9ee541ba-d0e4-4538-9089-a28fc8009398 (Autodesk Fusion 360 design; units mm, degrees)
Autodesk Fusion 360 part; units mm, degrees
note: some values were not read from the file. Set by a fixed rule: which sketch regions a step uses.
sketch "Sketch1" plane through (0, 0, 0) normal (0, 1, 0) x (1, 0, 0)
  circle A0 centre (0, 0) radius 6.35
  circle A1 centre (0, 0) radius 7.366
  circle A2 centre (0, 0) radius 5.2917
  circle A3 centre (0, 0) radius 5.967
  arc A4 (7.3471, -0.527) -> (-6.7515, -2.9454) centre (0, 0) ccw
  circle A5 centre (0, 0) radius 1.9844
  line L0 (0, 0) -> (7.366, 0) construction
  line L1 (0, 0) -> (-0.5201, -5.9443)
  line L2 (0, 0) -> (-1.0362, -5.8764)
  line L3 (0, 0) -> (-1.5444, -5.7637)
  line L4 (0, 0) -> (-2.0409, -5.6072)
  line L5 (0, 0) -> (-2.5218, -5.408)
  line L6 (0, 0) -> (-2.9835, -5.1676)
  line L7 (0, 0) -> (-3.4226, -4.8879)
  line L8 (-0.5201, -5.9443) -> (-0.0013, -5.9897) construction
  line L9 (-1.0362, -5.8764) -> (-0.0105, -6.0572) construction
  line L10 (-1.5444, -5.7637) -> (-0.0354, -6.168) construction
  line L11 (-2.0409, -5.6072) -> (-0.0836, -6.3196) construction
  line L12 (-2.5218, -5.408) -> (-0.1621, -6.5083) construction
  line L13 (-2.9835, -5.1676) -> (-0.2778, -6.7298) construction
  line L14 (-3.4226, -4.8879) -> (-0.4367, -6.9786) construction
  line L15 (0, 0) -> (-3.8355, -4.571)
  line L16 (-3.8355, -4.571) -> (-0.6444, -7.2487) construction
  line L17 (0, 0) -> (-4.2193, -4.2193)
  line L18 (-4.2193, -4.2193) -> (-0.9055, -7.5332) construction
  spline S0 degree 5 poles (-0.9055, -7.5332) (-0.8962, -7.5235) (-0.8778, -7.504) (-0.8503, -7.475) (-0.8141, -7.4367) (-0.7697, -7.3892) (-0.7263, -7.3419) (-0.6841, -7.2948) (-0.6432, -7.2478) (-0.6037, -7.2007) (-0.5658, -7.1536) (-0.5293, -7.1065) (-0.4942, -7.0596) (-0.4605, -7.0129) (-0.4281, -6.9665) (-0.3968, -6.9205) (-0.3669, -6.875) (-0.3381, -6.83) (-0.3106, -6.7855) (-0.2843, -6.7415) (-0.2594, -6.698) (-0.2358, -6.6552) (-0.2134, -6.613) (-0.1923, -6.5715) (-0.1725, -6.5308) (-0.1539, -6.4909) (-0.1364, -6.4518) (-0.1202, -6.4138) (-0.1051, -6.3767) (-0.0912, -6.3407) (-0.0784, -6.3058) (-0.0668, -6.2721) (-0.0562, -6.2397) (-0.0467, -6.2086) (-0.0383, -6.1789) (-0.0308, -6.1507) (-0.0242, -6.1241) (-0.0186, -6.0992) (-0.0139, -6.076) (-0.01, -6.0547) (-0.0069, -6.0353) (-0.0045, -6.018) (-0.0027, -6.0029) (-0.0013, -5.9903) (-0.0004, -5.9802) (0.0001, -5.9728) (0.0003, -5.9691) (0.0002, -5.9676) (0.0001, -5.9671) (0, -5.967) knots 0 0 0 0 0 0 0.022222 0.044444 0.066667 0.088889 0.111111 0.133333 0.155556 0.177778 0.2 0.222222 0.244444 0.266667 0.288889 0.311111 0.333333 0.355556 0.377778 0.4 0.422222 0.444444 0.466667 0.488889 0.511111 0.533333 0.555556 0.577778 0.6 0.622222 0.644444 0.666667 0.688889 0.711111 0.733333 0.755556 0.777778 0.8 0.822222 0.844444 0.866667 0.888889 0.911111 0.933333 0.955556 0.977778 1 1 1 1 1 1
  line L19 (-1.012, -7.6454) -> (-0.7989, -7.421)
  line L20 (0.0091, -5.9765) -> (-0.0091, -5.9576)
  line L21 (-0.0946, -6.3493) -> (0, 0)
  line L22 (0, 0) -> (-0.8866, -6.0377) construction
  line L23 (0, -5.967) -> (0, 0) construction
  spline S1 degree 5 poles (0, -5.967) (0, -5.9285) (0, -5.8556) (0, -5.7592) (0, -5.6519) (0, -5.5361) (0, -5.4448) (0, -5.3711) (0, -5.3187) (0, -5.2917) knots 0 0 0 0 0 0 0.2 0.4 0.6 0.8 1 1 1 1 1 1
  spline S2 degree 5 poles (-1.7155, -5.7151) (-1.7044, -5.6782) (-1.6834, -5.6084) (-1.6557, -5.516) (-1.6249, -5.4133) (-1.5916, -5.3024) (-1.5653, -5.215) (-1.5441, -5.1443) (-1.5291, -5.0941) (-1.5213, -5.0683) knots 0 0 0 0 0 0 0.2 0.4 0.6 0.8 1 1 1 1 1 1
  line L24 (0, -6.0408) -> (0, -5.8933)
  line L25 (0, -5.3433) -> (0, -5.24)
  line L26 (-1.7367, -5.7858) -> (-1.6943, -5.6445)
  line L27 (-1.5362, -5.1178) -> (-1.5064, -5.0188)
  spline S3 degree 5 poles (-1.2985, -7.4755) (-1.3045, -7.4635) (-1.3166, -7.4396) (-1.3346, -7.4039) (-1.3582, -7.3568) (-1.3871, -7.2985) (-1.4151, -7.2408) (-1.442, -7.1835) (-1.4676, -7.1267) (-1.4919, -7.0703) (-1.5147, -7.0142) (-1.5361, -6.9587) (-1.5562, -6.9036) (-1.5751, -6.8492) (-1.5928, -6.7954) (-1.6095, -6.7424) (-1.6251, -6.6902) (-1.6397, -6.6388) (-1.6533, -6.5883) (-1.6658, -6.5386) (-1.6772, -6.4899) (-1.6875, -6.442) (-1.6968, -6.3952) (-1.705, -6.3494) (-1.7123, -6.3046) (-1.7187, -6.2611) (-1.7242, -6.2187) (-1.7288, -6.1776) (-1.7326, -6.1377) (-1.7355, -6.0992) (-1.7377, -6.0622) (-1.7392, -6.0265) (-1.74, -5.9924) (-1.7401, -5.9599) (-1.7397, -5.9291) (-1.7388, -5.8999) (-1.7374, -5.8726) (-1.7357, -5.8471) (-1.7335, -5.8235) (-1.7311, -5.8019) (-1.7285, -5.7825) (-1.7258, -5.7652) (-1.7232, -5.7503) (-1.7209, -5.7378) (-1.7189, -5.7279) (-1.7173, -5.7206) (-1.7163, -5.717) (-1.7158, -5.7156) (-1.7156, -5.7152) (-1.7155, -5.7151) knots 0 0 0 0 0 0 0.022222 0.044444 0.066667 0.088889 0.111111 0.133333 0.155556 0.177778 0.2 0.222222 0.244444 0.266667 0.288889 0.311111 0.333333 0.355556 0.377778 0.4 0.422222 0.444444 0.466667 0.488889 0.511111 0.533333 0.555556 0.577778 0.6 0.622222 0.644444 0.666667 0.688889 0.711111 0.733333 0.755556 0.777778 0.8 0.822222 0.844444 0.866667 0.888889 0.911111 0.933333 0.955556 0.977778 1 1 1 1 1 1
  line L28 (-1.2286, -7.6136) -> (-1.3683, -7.3374)
  line L29 (-1.7269, -5.7215) -> (-1.7041, -5.7087)
  point P0 (-0.0946, -6.3493)
  point P1 (0, -5.2917)
  point P2 (-1.4668, -7.128)
  point P3 (-1.588, -6.8096)
  point P4 (-1.6687, -6.5255)
  point P5 (-1.7158, -6.2802)
  point P6 (-1.7368, -6.0768)
  point P7 (-1.7393, -5.9178)
  point P8 (-1.7313, -5.8046)
  point P9 (-1.7207, -5.7372)
  point P10 (-1.5213, -5.0683)
  dimension "d2" = 14.732
  dimension "id" = 10.5833
  dimension "BaseDiameter" = 11.9341
  dimension "d1" = 3.9688
  dimension "d34" = 5
  dimension "d35" = 5
  dimension "d36" = 5
  dimension "d37" = 5
  dimension "d38" = 5
  dimension "d39" = 5
  dimension "d41" = 0.5207
  dimension "d42" = 1.0414
  dimension "d43" = 1.5622
  dimension "d44" = 2.0829
  dimension "d45" = 2.6036
  dimension "d46" = 3.1243
  dimension "d47" = 3.6451
  dimension "d48" = 5
  dimension "d49" = 4.1658
  dimension "d50" = 5
  dimension "d51" = 4.6865
  dimension "d55" = 7.5
  dimension "d60" = 5
  constraint coincident A0.centre A1.centre
  constraint concentric A0 A2
  constraint coincident A1 A4.end
  constraint horizontal L0
  constraint coincident A4 L0.end
  constraint coincident A3 S0.end
  constraint coincident A3 L1.end
  constraint coincident A3 L2.end
  constraint coincident A3 L3.end
  constraint coincident A3 L4.end
  constraint coincident A3 L5.end
  constraint coincident A3 L6.end
  constraint coincident A3 L7.end
  constraint vertical A0.centre S0.end
  constraint tangent A3 L8
  constraint tangent A3 L9
  constraint tangent A3 L10
  constraint tangent A3 L11
  constraint tangent A3 L12
  constraint tangent A3 L13
  constraint tangent A3 L14
  constraint coincident A3 L15.end
  constraint tangent A3 L16
  constraint coincident A3 L17.end
  constraint tangent A3 L18
  constraint midpoint L18.end L19
  constraint midpoint S0.end L20
  constraint coincident A0 P0
  constraint coincident S0 P0
  constraint coincident P0 L21.start
  constraint coincident L23 P1
  constraint coincident A2 P1
  constraint coincident P1 S1.end
  constraint midpoint S0.end L24
  constraint midpoint P1 L25
  constraint symmetric S0.end L22 S2.start
  constraint symmetric L8.end L22 P9
  constraint symmetric L9.end L22 P8
  constraint symmetric L10.end L22 P7
  constraint symmetric L11.end L22 P6
  constraint symmetric L12.end L22 P5
  constraint symmetric L13.end L22 P4
  constraint symmetric L14.end L22 P3
  constraint symmetric L16.end L22 P2
  constraint symmetric L18.end L22 S3.start
  constraint symmetric L19.start L22 L28.start
  constraint symmetric L19.end L22 L28.end
  constraint symmetric L20.start L22 L29.start
  constraint symmetric L20.end L22 L29.end
  constraint symmetric L22 P1 P10
  constraint symmetric L22 L24.start L26.start
  constraint symmetric L22 L24.end L26.end
  constraint symmetric L22 L25.start L27.start
  constraint symmetric L22 L25.end L27.end
  constraint vertical L24
  constraint vertical L25
  measures "d2" diameter of A1
  measures "id" diameter of A2
  measures "BaseDiameter" diameter of A3
  measures "d1" diameter of A5
  measures "d34" angle of L1 L2
  measures "d35" angle of L2 L3
  measures "d36" angle of L3 L4
  measures "d37" angle of L4 L5
  measures "d38" angle of L5 L6
  measures "d39" angle of L6 L7
  measures "d41" distance of L1.end L8.end
  measures "d42" distance of L2.end L9.end
  measures "d43" distance of L3.end L10.end
  measures "d44" distance of L4.end L11.end
  measures "d45" distance of L5.end L12.end
  measures "d46" distance of L6.end L13.end
  measures "d47" distance of L7.end L14.end
  measures "d48" angle of L7 L15
  measures "d49" distance of L15.end L16.end
  measures "d50" angle of L15 L17
  measures "d51" distance of L17.end L18.end
  measures "d55" angle of L21 L22
  measures "d60" angle of L1 L23
extrude "Extrude1" add sketch "Sketch1" along normal blind 304.8 contours A0 A1 S0 S3 | A3 S0 L21 | A0 A3 L21 S3 | A2 A3 L21 S1 L24 L25 | A2 A3 L1 L21 | A2 A3 L3 S2 L26 L27 | A2 A3 L1 L2 | A2 A3 L2 L3 makes body 1
pattern_circular "C-Pattern2" count 12 over 360 about axis through (0, 1.75, 0) along (0, 1, 0) of bodies 1 makes body 2 at (1.3828, 101.6, 5.1078) makes body 3 at (3.7515, 101.6, 3.7321) makes body 4 at (5.1149, 101.6, 1.3563) makes body 5 at (5.1078, 101.6, -1.3828) makes body 6 at (3.7321, 101.6, -3.7515) makes body 7 at (1.3563, 101.6, -5.1149) makes body 8 at (-1.3828, 101.6, -5.1078) makes body 9 at (-3.7515, 101.6, -3.7321) makes body 10 at (-5.1149, 101.6, -1.3563) makes body 11 at (-5.1078, 101.6, 1.3828) makes body 12 at (-3.7321, 101.6, 3.7515)
extrude "Extrude2" add sketch "Sketch1" along normal blind 304.8 contours A2 A5 L17 L21 | A2 A5 L1 L21 | A2 A5 L1 L2 | A2 A5 L3 L4 | A2 A5 L4 L5 | A2 A5 L2 L3 | A2 A5 L15 L17 | A2 A5 L5 L6 | A2 A5 L7 L15 | A2 A5 L6 L7 bodies 1 2 3 4 5 6 7 8 9 10 11 12
ref_plane "WorkPlane1" through (6.2747, 152.4, -0.8261) normal (0.130526, 0, 0.991445) x (0.991445, 0, -0.130526)
fillet "Fillet1" [suppressed]
mirror "Mirror3" [suppressed]
pattern_circular "C-Pattern1" [suppressed]
equation "d = 0.5 in"
equation "OutsideDiameter = d2"
equation "PitchDiameter = d"
equation "id = PitchDiameter - 2 * ( PitchDiameter / TeethNumber )"
equation "BaseDiameter = PitchDiameter * cos(20 deg)"
equation "Length = 12 in"
equation "t = 12"
equation "ShaftDiameter = d1"
equation "TeethNumber = t"
equation "Pitch = 32"
equation "d30 = ( 1.25 * ( PitchDiameter / TeethNumber ) ) - ( PitchDiameter / TeethNumber )"
equation "Basecircum = PI * PitchDiameter * cos(20 deg)"
equation "d41 = Basecircum * 5 / 360"
equation "d42 = Basecircum * 10 / 360"
equation "d43 = Basecircum * 15 / 360"
equation "d44 = Basecircum * 20 / 360"
equation "d45 = Basecircum * 25 / 360"
equation "d46 = Basecircum * 30 / 360"
equation "d47 = Basecircum * 35 / 360"
equation "d49 = Basecircum * 40 / 360"
equation "d51 = Basecircum * 45 / 360"
equation "d55 = ( 360 / ( 4 * TeethNumber ) ) * 1 deg"
